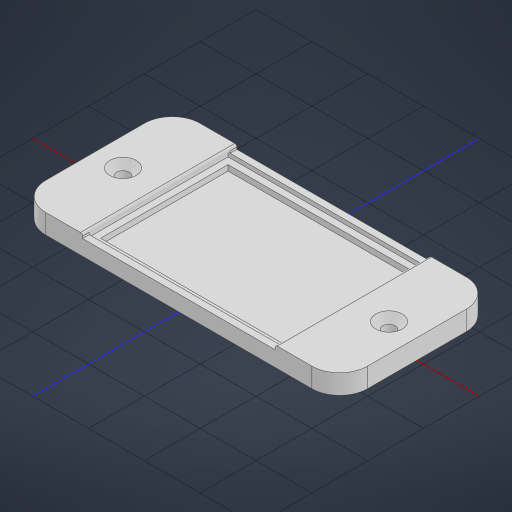
# Autodesk Inventor part: PCB_Holder_B
Saved by Autodesk Inventor 2023.2 (Build 272271030, 271C)
## iProperties
Created: 2023-05-22
Part Number: PCB_Holder_B
Material: Generisch
Document SubType Name: Modeling
Designer: Stefan
Mass: 26.6057 g
Surface Area: 158.192 cm^2
Volume: 26.6057 cm^3
Density: 1 g/cm^3
Appearance: Vorgabe
Author: Stefan
Autodesk Inventor part; units mm, degrees
ref_plane "YZ Plane" through (0, 0, 0) normal (1, 0, 0) x (0, 1, 0)
ref_plane "XZ Plane" through (0, 0, 0) normal (0, 1, 0) x (-1, 0, 0)
ref_plane "XY Plane" through (0, 0, 0) normal (0, 0, 1) x (1, 0, 0)
sketch "Skizze1" plane through (0, 0, 0) normal (0, 1, 0) x (-1, 0, 0)
  line L0 (35.25, -25.25) -> (-35.25, -25.25)
  line L1 (-35.25, -25.25) -> (-35.25, 25.25)
  line L2 (-35.25, 25.25) -> (35.25, 25.25)
  line L3 (35.25, 25.25) -> (35.25, -25.25)
  line L4 (35.25, -25.25) -> (-35.25, 25.25) construction
  line L5 (-35.25, -25.25) -> (35.25, 25.25) construction
  line L6 (37.65, -27.65) -> (-37.65, -27.65)
  line L7 (-37.65, -27.65) -> (-37.65, 27.65)
  line L8 (-37.65, 27.65) -> (37.65, 27.65)
  line L9 (37.65, 27.65) -> (37.65, -27.65)
  line L10 (32.85, -22.85) -> (-32.85, -22.85)
  line L11 (-32.85, -22.85) -> (-32.85, 22.85)
  line L12 (-32.85, 22.85) -> (32.85, 22.85)
  line L13 (32.85, 22.85) -> (32.85, -22.85)
  line L14 (47.65, -27.65) -> (37.65, -27.65)
  line L15 (37.65, 27.65) -> (47.65, 27.65)
  circle A0 centre (47.65, 0) radius 2
  line L16 (-37.65, -27.65) -> (-47.65, -27.65)
  line L17 (-37.65, 27.65) -> (-47.65, 27.65)
  circle A1 centre (-47.65, 0) radius 2
  arc A2 (-47.65, 27.65) -> (-57.65, 17.65) centre (-47.65, 17.65) ccw
  arc A3 (-57.65, -17.65) -> (-47.65, -27.65) centre (-47.65, -17.65) ccw
  line L18 (-57.65, 17.65) -> (-57.65, -17.65)
  arc A4 (57.65, 17.65) -> (47.65, 27.65) centre (47.65, 17.65) ccw
  arc A5 (47.65, -27.65) -> (57.65, -17.65) centre (47.65, -17.65) ccw
  line L19 (57.65, 17.65) -> (57.65, -17.65)
  point P0 (0, 0)
  point P1 (86.5572, 0)
  point P2 (-87.7335, 0)
  point P3 (57.65, 0)
  point P4 (-57.65, 0)
  dimension "d0" = 70.5
  dimension "d1" = 50.5
  dimension "d2" = 2.4
  dimension "d3" = 2.4
  dimension "d4" = 4
  dimension "d7" = 4
  dimension "d28" = 20
  dimension "d29" = 20
  dimension "d30" = 10
  dimension "d31" = 10
  dimension "d32" = 10
  dimension "d33" = 10
  constraints: 40 end point, 9 point on circle, 8 tangent, 6 centre point, 6 parallel, 4 collinear, 4 midpoint, 3 perpendicular, 2 equal radius, 2 horizontal alignment, 2 vertical, 1 horizontal, 6 other
  measures "d0" distance of L1.end L2.end
  measures "d1" distance of L0.end L1.end
  measures "d2" distance between parallel lines of L3 L9
  measures "d3" distance between parallel lines of L13 L3
  measures "d4" diameter of A0
  measures "d7" diameter of A1
  measures "d28" distance between parallel lines of L9 L19
  measures "d29" distance between parallel lines of L18 L7
  measures "d30" radius of A4
  measures "d31" distance from line of L9 A0.centre
  measures "d32" distance from line of A1.centre L7
  measures "d33" radius of A2
extrude "Extrusion1" add sketch "Skizze1" against normal blind 2 contours L0 L1 L2 L3 | L6 L7 L8 L9 | L9 L15 A4 L19 A5 L14 | L16 A3 L18 A2 L17 L7 | L10 L11 L12 L13
extrude "Extrusion2" add sketch "Skizze1" along normal blind 5 contours L6 L7 L8 L9 | L9 L15 A4 L19 A5 L14 | L16 A3 L18 A2 L17 L7
extrude "Extrusion3" add sketch "Skizze1" along normal blind 2 contours L0 L1 L2 L3
sketch "Skizze2" plane through (0, 0, 0) normal (0, 0, 1) x (1, 0, 0)
  line L0 (32.85, 0) -> (32.85, 2) projected
  line L1 (32.85, 2) -> (35.25, 2) projected
  line L2 (35.25, 2) -> (35.25, 5) projected
  line L3 (35.25, 5) -> (45.65, 5) projected
  line L4 (45.65, 5) -> (45.65, -2) projected
  line L5 (45.65, -2) -> (-45.65, -2) projected
  line L6 (-45.65, -2) -> (-45.65, 5) projected
  line L7 (-45.65, 5) -> (-35.25, 5) projected
  line L8 (-35.25, 5) -> (-35.25, 2) projected
  line L9 (-35.25, 2) -> (-32.85, 2) projected
  line L10 (-32.85, 2) -> (-32.85, 0) projected
  line L11 (-32.85, 0) -> (32.85, 0) projected
  line L12 (-57.65, 5) -> (-49.65, 5) projected
  line L13 (-49.65, 5) -> (-49.65, -2) projected
  line L14 (-49.65, -2) -> (-57.65, -2) projected
  line L15 (49.65, 5) -> (57.65, 5) projected
  line L16 (57.65, -2) -> (49.65, -2) projected
  line L17 (49.65, -2) -> (49.65, 5) projected
  arc A0 (-35.25, 3.5) -> (-35.25, 5) centre (-35.25, 4.25) ccw
  arc A1 (35.25, 5) -> (35.25, 3.5) centre (35.25, 4.25) ccw
  line L18 (-35.25, 5) -> (-35.25, 3.5)
  line L19 (35.25, 5) -> (35.25, 3.5)
  line L20 (-34.5, 4.25) -> (-34.5, 3.5)
  line L21 (-35.25, 2) -> (35.25, 2) projected
  line L22 (35.25, 2) -> (35.25, 5) projected
  line L23 (-35.25, 3.5) -> (35.25, 3.5)
  line L24 (-35.25, 5) -> (35.25, 5)
  line L25 (47.65, 5) -> (-47.65, 5) projected
  line L26 (34.5, 4.25) -> (34.5, 3.5)
  line L27 (-57.65, -2) -> (-57.65, 5) projected
  line L28 (57.65, 5) -> (57.65, -2) projected
  point P0 (0, 0)
  point P1 (39.5, 3.725)
  point P2 (39.8372, 3.6239)
  point P3 (-39.5, 3.725)
  point P4 (-39.8372, 3.6239)
  dimension "d14" = 1.5
  dimension "d15" = 1.5
  constraints: 12 end point, 6 point on circle, 4 tangent, 2 centre point, 2 collinear, 2 midpoint, 2 perpendicular, 2 point on line, 1 vertical
  measures "d14" distance from line of L18.end L9
  measures "d15" distance from line of L19.end L1
extrude "Extrusion4" add sketch "Skizze2" along normal mid plane 50.5 contours A1 L2 | L8 A0
extrude "Extrusion5" cut sketch "Skizze2" along normal through all both and the other way through all contours A1 L26 L23 L20 A0 L24
sketch "Skizze3" plane through (0, 5, 0) normal (0, 1, 0) x (1, 0, 0)
  circle A0 centre (-47.65, 0) radius 2 projected
  circle A1 centre (47.65, 0) radius 2 projected
  point P0 (0, 0)
  constraints: 2 coincident
hole "Bohrung1" at (-47.65, 5, 0) at (47.65, 5, 0) direction (0, -1, 0) diameter 4.5 depth 6 countersink diameter 9.4 countersink angle 90 clearance for "Flachkopfsenkschraube DIN EN ISO 2009" size "M4" standard "DIN"
equation "\"d7\" = d4"
equation "\"d29\" = d28"
equation "\"d32\" = d31"
equation "\"d33\" = d30"
equation "\"d15\" = d14"
